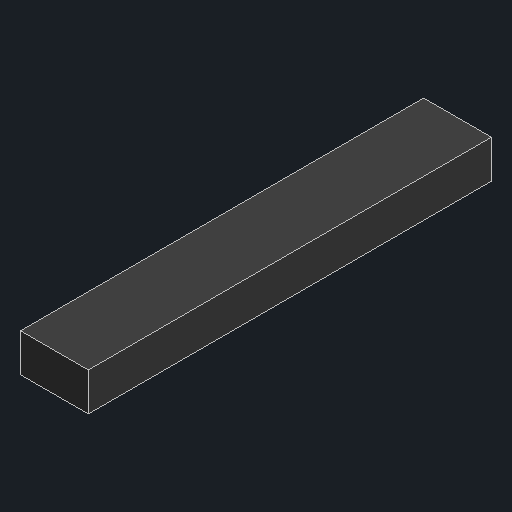
# Autodesk Inventor part: sample
Saved by Autodesk Inventor 2026.1 (Build 301233020, 233B)
## iProperties
Created: 2025-12-10
Part Number: sample
Material: 고무, 검은색
Document SubType Name: Modeling
Designer: jaewook
Density: 0.93 g/cm^3
Appearance: 고무 - 검은색
Author: jaewook
Autodesk Inventor part; units mm, degrees
ref_plane "YZ Plane" through (0, 0, 0) normal (1, 0, 0) x (0, 1, 0)
ref_plane "XZ Plane" through (0, 0, 0) normal (0, 1, 0) x (-1, 0, 0)
ref_plane "XY Plane" through (0, 0, 0) normal (0, 0, 1) x (1, 0, 0)
sketch "스케치1" plane through (0, 0, 0) normal (0, 1, 0) x (-1, 0, 0)
  line L0 (88.0955, 15.6086) -> (88.0955, 68.8243)
  line L1 (97.5955, 15.6086) -> (88.0955, 15.6086)
  line L2 (97.5955, 68.8243) -> (97.5955, 15.6086)
  line L3 (88.3955, 69.1243) -> (88.3955, 15.9086)
  line L4 (88.3955, 15.9086) -> (97.2955, 15.9086)
  line L5 (97.2955, 15.9086) -> (97.2955, 69.1243)
  line L6 (97.5955, 68.8243) -> (88.0955, 68.8243)
  point P0 (0, 0)
  point P1 (86.7957, 68.8243)
  point P2 (97.2955, 68.8243)
  point P3 (88.3955, 68.8243)
  point P4 (97.2955, 68.8243)
  point P5 (88.3955, 68.8243)
  dimension "d0" = 0.3
  constraints: 14 end point, 2 point on line, 1 horizontal, 2 other
  measures "d0" distance between parallel lines of L0 L3
extrude "돌출1" add sketch "스케치1" along normal blind 5 contours L6 L5 L4 L3
